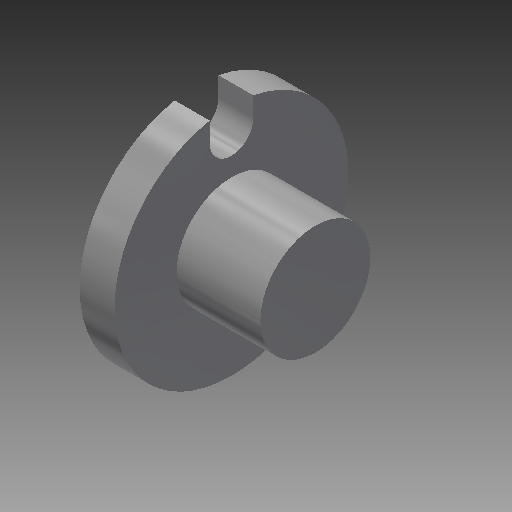
# Autodesk Inventor part: Pulley Shaft
Saved by Autodesk Inventor 2017 (Build 210135000, 135)
## iProperties
Created: 2012-08-06
Part Number: Pulley Shaft
Material: Steel
Document SubType Name: Modeling
Designer: John
Mass: 13.0314 g
Surface Area: 11.3717 cm^2
Volume: 1.66006 cm^3
Density: 7.85 g/cm^3
Appearance: Steel
Author: John
Autodesk Inventor part; units mm, degrees
ref_plane "YZ Plane" through (0, 0, 0) normal (1, 0, 0) x (0, 1, 0)
ref_plane "XZ Plane" through (0, 0, 0) normal (0, 1, 0) x (-1, 0, 0)
ref_plane "XY Plane" through (0, 0, 0) normal (0, 0, 1) x (1, 0, 0)
sketch "Sketch1" plane through (0, 0, 0) normal (1, 0, 0) x (0, 1, 0)
  circle A0 centre (0, 0) radius 8.509
  dimension "d1" = 17.018
  constraints: 1 centre point, 1 coincident
  measures "d1" diameter of A0
extrude "Extrusion1" add sketch "Sketch1" along normal blind 2.54
sketch "Sketch2" plane through (2.54, 0, 0) normal (1, 0, 0) x (0, 0, -1)
  circle A0 centre (0, 0) radius 8.509 projected
  circle A1 centre (0, 0) radius 4.0005
  dimension "d5" = 8.001
  constraints: 1 centre point, 1 coincident
  measures "d5" diameter of A1
extrude "Extrusion2" add sketch "Sketch2" along normal blind 6.096 contours A1
sketch "Sketch3" plane through (0, 0, 0) normal (-1, 0, 0) x (0, 0, 1)
  circle A0 centre (0, 0) radius 8.509 projected
  circle A1 centre (6.9342, 0) radius 1.5875
  line L0 (6.9342, -1.5875) -> (8.3596, -1.5875)
  line L1 (6.9342, 1.5875) -> (8.3596, 1.5875)
  line L2 (6.9342, 0) -> (0, 0)
  dimension "d8" = 6.9342
  dimension "d9" = 3.175
  constraints: 6 end point, 4 point on circle, 2 parallel, 2 tangent, 1 centre point, 1 horizontal
  measures "d8" distance of L2.start L2.end
  measures "d9" diameter of A1
extrude "Extrusion3" cut sketch "Sketch3" against normal through all contours A0 A1 L1 | L0 A1 A0 | A1 A0 | A0 A1
body "Solid1"
